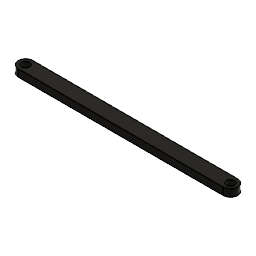
Australia Brace Bar (Autodesk Fusion 360 design; units mm, degrees)
part number: 2026-04-20-17-15-41-321
Autodesk Fusion 360 part; units mm, degrees
note: some values were not read from the file. Set by a fixed rule: which sketch regions a step uses.
sketch "Sketch1" plane through (0, 0, 0) normal (0, 1, 0) x (1, 0, 0)
  line L0 (-42.5, 0) -> (42.5, 0)
  line L1 (-42.5, 3) -> (42.5, 3)
  line L2 (42.5, -3) -> (-42.5, -3)
  circle A0 centre (-42.5, 0) radius 1.65
  circle A1 centre (-42.5, 0) radius 3
  circle A2 centre (42.5, 0) radius 3
  circle A3 centre (42.5, 0) radius 1.65
  dimension "d1" = 85
  dimension "d8" = 3.3
  dimension "d9" = 6
  dimension "d10" = 3.3
  constraint midpoint L0 origin
  constraint horizontal L0
  constraint horizontal L1
  constraint horizontal L2
  constraint coincident L0.start A0.centre
  constraint concentric A0 A1
  constraint tangent L2 A1
  constraint coincident A1 L1.start
  constraint coincident A1 L2.end
  constraint coincident L0.end A2.centre
  constraint concentric A2 A3
  constraint coincident A2 L1.end
  constraint coincident A2 L2.start
  measures "d1" distance of L0.start L0.end
  measures "d8" diameter of A0
  measures "d9" diameter of A2
  measures "d10" diameter of A3
extrude "Extrude1" add sketch "Sketch1" along normal blind 3
